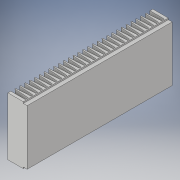
# Autodesk Inventor part: chladic
Saved by Autodesk Inventor 2019 (Build 230136000, 136)
## iProperties
Created: 2021-01-08
Part Number: chladic
Material: Všeobecné
Document SubType Name: Modeling
Designer: Pokor
Density: 1 g/cm^3
Appearance: Výchozí
Author: Pokor
Autodesk Inventor part; units mm, degrees
ref_plane "YZ Plane" through (0, 0, 0) normal (1, 0, 0) x (0, 1, 0)
ref_plane "XZ Plane" through (0, 0, 0) normal (0, 1, 0) x (-1, 0, 0)
ref_plane "XY Plane" through (0, 0, 0) normal (0, 0, 1) x (1, 0, 0)
sketch "Náčrt1" plane through (0, 0, 0) normal (0, 1, 0) x (-1, 0, 0)
  line L0 (0, 0) -> (40, 0)
  line L1 (40, 0) -> (40, -6)
  line L2 (40, -6) -> (10, -6)
  line L3 (0, 0) -> (0, -15)
  arc A0 (40, -15) -> (38.8258, -13.7523) centre (38.75, -15) ccw
  line L4 (10, -6) -> (10, -12)
  line L5 (38.8258, -13.7523) -> (10, -12)
  line L6 (0, -15) -> (40, -15)
  dimension "d0" = 40
  dimension "d1" = 6
  dimension "d4" = 2.5
  dimension "d5" = 10
  dimension "d8" = 15
  dimension "d9" = 6
  dimension "d10" = 93.479
  dimension "d12" = 15
  constraints: 16 end point, 2 horizontal, 2 perpendicular, 2 point on circle, 2 tangent, 2 vertical, 1 centre point
  measures "d0" distance of L0.start L0.end
  measures "d1" distance of L0.end L1.end
  measures "d4" diameter of A0
  measures "d5" distance between parallel lines of L4 L3
  measures "d8" distance from line of L0 A0.centre
  measures "d9" distance of L2.end L4.end
  measures "d10" angle of L4 L5
  measures "d12" distance between parallel lines of L0 L6
extrude "Vysunutí1" add sketch "Náčrt1" along normal blind 120
sketch "Náčrt2" plane through (0, 120, 0) normal (0, 1, 0) x (1, 0, 0)
  line L0 (-40, 0) -> (0, 0) projected
  line L1 (0, 0) -> (0, 15) projected
  line L2 (0, 15) -> (-40, 15) projected
  arc A0 (-40, 15) -> (-38.8258, 13.7523) centre (-38.75, 15) ccw projected
  line L3 (-38.8258, 13.7523) -> (-10, 12) projected
  line L4 (-10, 12) -> (-10, 6) projected
  line L5 (-10, 6) -> (-40, 6) projected
  line L6 (-40, 6) -> (-40, 0) projected
  line L7 (0, 15) -> (0, 25)
  line L8 (0, 25) -> (-40, 25)
  line L9 (-10, 18) -> (-38.8258, 16.2477)
  line L10 (-10, 22) -> (-38.8258, 23.7523)
  arc A1 (-40, 25) -> (-38.8258, 23.7523) centre (-38.75, 25) ccw
  line L11 (-40, 6) -> (-40, 0) projected
  line L12 (-10, 18) -> (-10, 22)
  line L13 (-40, 15) -> (0, 15)
  arc A2 (-38.8258, 16.2477) -> (-40, 15) centre (-38.75, 15) ccw
  line L14 (0, 15) -> (-40, 15) projected
  dimension "d15" = 1.25
  dimension "d16" = 2.5
  dimension "d18" = 10
  dimension "d19" = 10
  dimension "d20" = 10
  dimension "d21" = 86.521
  dimension "d22" = 86.521
  dimension "d24" = 1.25
  constraints: 13 end point, 4 point on circle, 4 tangent, 3 point on line, 2 centre point, 2 equal length, 2 vertical, 1 perpendicular
  measures "d15" radius of A0
  measures "d16" diameter of A1
  measures "d18" distance between parallel lines of L8 L2
  measures "d19" distance between parallel lines of L1 L4
  measures "d20" distance between parallel lines of L7 L12
  measures "d21" angle of L10 L12
  measures "d22" angle of L9 L12
  measures "d24" radius of A2
extrude "Vysunutí2" add sketch "Náčrt2" against normal blind 120 contours L2 A2 L9 L12 L10 A1 L8 L7
pattern_linear "Obdélníkové pole1" count 27 spacing 10 along (0, 0, -1) of "Vysunutí2"
sketch "Náčrt3" plane through (0, 120, 0) normal (0, 1, 0) x (1, 0, 0)
  line L0 (-40, 0) -> (0, 0) projected
  line L1 (0, 0) -> (0, 285) projected
  line L2 (-38.8258, 263.7523) -> (-10, 262) projected
  line L3 (-10, 262) -> (-10, 258) projected
  line L4 (-10, 258) -> (-38.8258, 256.2477) projected
  arc A0 (-38.8258, 256.2477) -> (-38.8258, 253.7523) centre (-38.75, 255) ccw projected
  line L5 (-38.8258, 253.7523) -> (-10, 252) projected
  line L6 (-10, 252) -> (-10, 248) projected
  line L7 (-10, 248) -> (-38.8258, 246.2477) projected
  arc A1 (-38.8258, 246.2477) -> (-38.8258, 243.7523) centre (-38.75, 245) ccw projected
  line L8 (-38.8258, 243.7523) -> (-10, 242) projected
  line L9 (-10, 242) -> (-10, 238) projected
  line L10 (-10, 238) -> (-38.8258, 236.2477) projected
  arc A2 (-38.8258, 236.2477) -> (-38.8258, 233.7523) centre (-38.75, 235) ccw projected
  line L11 (-38.8258, 233.7523) -> (-10, 232) projected
  line L12 (-10, 232) -> (-10, 228) projected
  line L13 (-10, 228) -> (-38.8258, 226.2477) projected
  arc A3 (-38.8258, 226.2477) -> (-38.8258, 223.7523) centre (-38.75, 225) ccw projected
  line L14 (-38.8258, 223.7523) -> (-10, 222) projected
  line L15 (-10, 222) -> (-10, 218) projected
  line L16 (-10, 218) -> (-38.8258, 216.2477) projected
  arc A4 (-38.8258, 216.2477) -> (-38.8258, 213.7523) centre (-38.75, 215) ccw projected
  line L17 (-38.8258, 213.7523) -> (-10, 212) projected
  line L18 (-10, 212) -> (-10, 208) projected
  line L19 (-10, 208) -> (-38.8258, 206.2477) projected
  arc A5 (-38.8258, 206.2477) -> (-38.8258, 203.7523) centre (-38.75, 205) ccw projected
  line L20 (-38.8258, 203.7523) -> (-10, 202) projected
  line L21 (-10, 202) -> (-10, 198) projected
  line L22 (-10, 198) -> (-38.8258, 196.2477) projected
  arc A6 (-38.8258, 196.2477) -> (-38.8258, 193.7523) centre (-38.75, 195) ccw projected
  line L23 (-38.8258, 193.7523) -> (-10, 192) projected
  line L24 (-10, 192) -> (-10, 188) projected
  line L25 (-10, 188) -> (-38.8258, 186.2477) projected
  arc A7 (-38.8258, 186.2477) -> (-38.8258, 183.7523) centre (-38.75, 185) ccw projected
  line L26 (-38.8258, 183.7523) -> (-10, 182) projected
  line L27 (-10, 182) -> (-10, 178) projected
  line L28 (-10, 178) -> (-38.8258, 176.2477) projected
  arc A8 (-38.8258, 176.2477) -> (-38.8258, 173.7523) centre (-38.75, 175) ccw projected
  line L29 (-38.8258, 173.7523) -> (-10, 172) projected
  line L30 (-10, 172) -> (-10, 168) projected
  line L31 (-10, 168) -> (-38.8258, 166.2477) projected
  arc A9 (-38.8258, 166.2477) -> (-38.8258, 163.7523) centre (-38.75, 165) ccw projected
  line L32 (-38.8258, 163.7523) -> (-10, 162) projected
  line L33 (-10, 162) -> (-10, 158) projected
  line L34 (-10, 158) -> (-38.8258, 156.2477) projected
  arc A10 (-38.8258, 156.2477) -> (-38.8258, 153.7523) centre (-38.75, 155) ccw projected
  line L35 (-38.8258, 153.7523) -> (-10, 152) projected
  line L36 (-10, 152) -> (-10, 148) projected
  line L37 (-10, 148) -> (-38.8258, 146.2477) projected
  arc A11 (-38.8258, 146.2477) -> (-38.8258, 143.7523) centre (-38.75, 145) ccw projected
  line L38 (-38.8258, 143.7523) -> (-10, 142) projected
  line L39 (-10, 142) -> (-10, 138) projected
  line L40 (-10, 138) -> (-38.8258, 136.2477) projected
  arc A12 (-38.8258, 136.2477) -> (-38.8258, 133.7523) centre (-38.75, 135) ccw projected
  line L41 (-38.8258, 133.7523) -> (-10, 132) projected
  line L42 (-10, 132) -> (-10, 128) projected
  line L43 (-10, 128) -> (-38.8258, 126.2477) projected
  arc A13 (-38.8258, 126.2477) -> (-38.8258, 123.7523) centre (-38.75, 125) ccw projected
  line L44 (-38.8258, 123.7523) -> (-10, 122) projected
  line L45 (-10, 122) -> (-10, 118) projected
  line L46 (-10, 118) -> (-38.8258, 116.2477) projected
  arc A14 (-38.8258, 116.2477) -> (-38.8258, 113.7523) centre (-38.75, 115) ccw projected
  line L47 (-38.8258, 113.7523) -> (-10, 112) projected
  line L48 (-10, 112) -> (-10, 108) projected
  line L49 (-10, 108) -> (-38.8258, 106.2477) projected
  arc A15 (-38.8258, 106.2477) -> (-38.8258, 103.7523) centre (-38.75, 105) ccw projected
  line L50 (-38.8258, 103.7523) -> (-10, 102) projected
  line L51 (-10, 102) -> (-10, 98) projected
  line L52 (-10, 98) -> (-38.8258, 96.2477) projected
  arc A16 (-38.8258, 96.2477) -> (-38.8258, 93.7523) centre (-38.75, 95) ccw projected
  line L53 (-38.8258, 93.7523) -> (-10, 92) projected
  line L54 (-10, 92) -> (-10, 88) projected
  line L55 (-10, 88) -> (-38.8258, 86.2477) projected
  arc A17 (-38.8258, 86.2477) -> (-38.8258, 83.7523) centre (-38.75, 85) ccw projected
  line L56 (-38.8258, 83.7523) -> (-10, 82) projected
  line L57 (-10, 82) -> (-10, 78) projected
  line L58 (-10, 78) -> (-38.8258, 76.2477) projected
  arc A18 (-38.8258, 76.2477) -> (-38.8258, 73.7523) centre (-38.75, 75) ccw projected
  line L59 (-38.8258, 73.7523) -> (-10, 72) projected
  line L60 (-10, 72) -> (-10, 68) projected
  line L61 (-10, 68) -> (-38.8258, 66.2477) projected
  arc A19 (-38.8258, 66.2477) -> (-38.8258, 63.7523) centre (-38.75, 65) ccw projected
  line L62 (-38.8258, 63.7523) -> (-10, 62) projected
  line L63 (-10, 62) -> (-10, 58) projected
  line L64 (-10, 58) -> (-38.8258, 56.2477) projected
  arc A20 (-38.8258, 56.2477) -> (-38.8258, 53.7523) centre (-38.75, 55) ccw projected
  line L65 (-38.8258, 53.7523) -> (-10, 52) projected
  line L66 (-10, 52) -> (-10, 48) projected
  line L67 (-10, 48) -> (-38.8258, 46.2477) projected
  arc A21 (-38.8258, 46.2477) -> (-38.8258, 43.7523) centre (-38.75, 45) ccw projected
  line L68 (-38.8258, 43.7523) -> (-10, 42) projected
  line L69 (-10, 42) -> (-10, 38) projected
  line L70 (-10, 38) -> (-38.8258, 36.2477) projected
  arc A22 (-38.8258, 36.2477) -> (-38.8258, 33.7523) centre (-38.75, 35) ccw projected
  line L71 (-38.8258, 33.7523) -> (-10, 32) projected
  line L72 (-10, 32) -> (-10, 28) projected
  line L73 (-10, 28) -> (-38.8258, 26.2477) projected
  arc A23 (-38.8258, 26.2477) -> (-38.8258, 23.7523) centre (-38.75, 25) ccw projected
  line L74 (-38.8258, 23.7523) -> (-10, 22) projected
  line L75 (-10, 22) -> (-10, 18) projected
  line L76 (-10, 18) -> (-38.8258, 16.2477) projected
  arc A24 (-38.8258, 16.2477) -> (-38.8258, 13.7523) centre (-38.75, 15) ccw projected
  line L77 (-38.8258, 13.7523) -> (-10, 12) projected
  line L78 (-10, 12) -> (-10, 6) projected
  line L79 (-10, 6) -> (-40, 6) projected
  line L80 (-40, 6) -> (-40, 0) projected
  line L81 (0, 300) -> (-40, 300)
  line L82 (-38.8258, 263.7523) -> (-10, 262) projected
  line L83 (-10, 262) -> (-10, 258) projected
  line L84 (-40, 300) -> (-40, 294)
  line L85 (-40, 294) -> (-10, 294)
  line L86 (-38.8258, 273.7523) -> (-10, 272) projected
  line L87 (-10, 272) -> (-10, 268) projected
  line L88 (-10, 268) -> (-38.8258, 266.2477) projected
  arc A25 (-38.8258, 266.2477) -> (-38.8258, 263.7523) centre (-38.75, 265) ccw projected
  line L89 (0, 285) -> (-40, 285) projected
  arc A26 (-40, 285) -> (-38.8258, 283.7523) centre (-38.75, 285) ccw projected
  line L90 (-38.8258, 283.7523) -> (-10, 282) projected
  line L91 (-10, 282) -> (-10, 278) projected
  line L92 (-10, 278) -> (-38.8258, 276.2477) projected
  arc A27 (-38.8258, 276.2477) -> (-38.8258, 273.7523) centre (-38.75, 275) ccw projected
  line L93 (-10, 288) -> (-38.8258, 286.2477)
  line L94 (0, 285) -> (-40, 285) projected
  arc A28 (-38.8258, 286.2477) -> (-40, 285) centre (-38.75, 285) ccw
  line L95 (-10, 288) -> (-10, 294)
  line L96 (-10, 282) -> (-10, 278) projected
  line L97 (0, 285) -> (0, 0) projected
  line L98 (0, 300) -> (0, 285)
  arc A29 (-40, 285) -> (-38.8258, 283.7523) centre (-38.75, 285) ccw projected
  line L99 (0, 285) -> (-40, 285)
  point P0 (0, 265)
  dimension "d30" = 1.25
  dimension "d33" = 40
  dimension "d38" = 6
  dimension "d39" = 30
  dimension "d49" = 15
  dimension "d50" = 10
  constraints: 14 end point, 2 point on circle, 1 centre point, 1 coincident, 1 collinear, 1 parallel, 1 perpendicular, 1 tangent, 1 vertical
  measures "d30" radius of A0
  measures "d33" distance of L81.start L81.end
  measures "d38" distance of L81.end L84.end
  measures "d39" distance of L84.end L85.end
  measures "d49" distance between parallel lines of L81 L89
  measures "d50" distance between parallel lines of L1 L95
extrude "Vysunutí3" add sketch "Náčrt3" against normal blind 120 contours L89 A28 L93 L95 L85 L84 L81 L98
sketch "Náčrt4" plane through (-40, 0, 0) normal (0, 0, 1) x (1, 0, 0)
  line L0 (40, 0) -> (40, 120) projected
  line L1 (40, 0) -> (32, 0)
  line L2 (32, 0) -> (32, 3)
  line L3 (32, 3) -> (40, 3)
  line L4 (40, 3) -> (40, 0)
  line L5 (0, 120) -> (40, 120) projected
  line L6 (40, 120) -> (32, 120)
  line L7 (32, 120) -> (32, 117)
  line L8 (32, 117) -> (40, 117)
  line L9 (40, 117) -> (40, 120)
  dimension "d42" = 3
  dimension "d45" = 8
  dimension "d53" = 8
  dimension "d54" = 3
  constraints: 16 end point, 4 parallel, 2 horizontal, 2 perpendicular
  measures "d42" distance of L1.end L2.end
  measures "d45" distance between parallel lines of L0 L2
  measures "d53" distance of L7.end L8.end
  measures "d54" distance between parallel lines of L8 L5
extrude "Vysunutí6" cut sketch "Náčrt4" against normal blind 300
equation "\"d9\" = d1"
equation "\"d12\" = d8"
equation "\"d16\" = 2 * d15"
equation "\"d20\" = d19"
equation "\"d22\" = d21"
